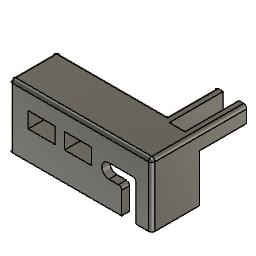
cordnew v7 (Autodesk Fusion 360 design; units mm, degrees)
Autodesk Fusion 360 part; units mm, degrees
sketch "Sketch1" plane through (0, 0, 0) normal (0, 1, 0) x (1, 0, 0)
  line L0 (0, 0) -> (90, 0)
  line L1 (90, 0) -> (90, -40)
  line L2 (90, -40) -> (0, -40)
  line L3 (0, -40) -> (0, 0)
  dimension "d1" = 90
  dimension "d2" = 40
  constraint horizontal L0
  constraint vertical L1
  constraint horizontal L2
  constraint vertical L3
  constraint coincident L0.start L3.end
  measures "d1" distance of L0.start L0.end
  measures "d2" distance of L0.end L1.end
extrude "Extrude1" add sketch "Sketch1" along normal blind 30
sketch "Sketch2" plane through (0, 30, 0) normal (0, 1, 0) x (-1, 0, 0)
  line L0 (0, 40) -> (-90, 40)
  line L1 (-90, 40) -> (-90, 0)
  line L2 (-90, 0) -> (0, 0)
  line L3 (0, 0) -> (0, 40)
  line L4 (-85, 0) -> (-5, 0)
  line L5 (-5, 0) -> (-5, 35)
  line L6 (-5, 35) -> (-85, 35)
  line L7 (-85, 35) -> (-85, 0)
  constraint horizontal L4
  constraint vertical L5
  constraint horizontal L6
  constraint vertical L7
  constraint coincident L2 L4.start
extrude "Extrude2" cut sketch "Sketch2" against normal blind 25 contours L2 L4 L5 L6 L7
sketch "Sketch3" plane through (0, 0, 0) normal (-1, 0, 0) x (0, -1, 0)
  line L0 (0, 0) -> (0, 40)
  line L1 (0, 40) -> (-30, 40)
  line L2 (-30, 40) -> (-30, 0)
  line L3 (-30, 0) -> (0, 0)
  line L4 (-25, 0) -> (-5, 0)
  line L5 (-5, 0) -> (-5, 10)
  line L6 (-5, 10) -> (-25, 10)
  line L7 (-25, 10) -> (-25, 0)
  constraint horizontal L4
  constraint vertical L5
  constraint horizontal L6
  constraint vertical L7
  constraint coincident L3 L4.start
extrude "Extrude3" cut sketch "Sketch3" against normal blind 5 contours L3 L4 L5 L6 L7
sketch "Sketch4" plane through (0, 30, 0) normal (0, 1, 0) x (-1, 0, 0)
  line L0 (-85, 0) -> (-85, 35)
  line L1 (-85, 35) -> (-5, 35)
  line L2 (-5, 35) -> (-5, 0)
  line L3 (-5, 0) -> (0, 0)
  line L4 (0, 0) -> (0, 40)
  line L5 (0, 40) -> (-90, 40)
  line L6 (-90, 40) -> (-90, 0)
  line L7 (-90, 0) -> (-85, 0)
  line L8 (-90, 40) -> (-70, 40)
  line L9 (-70, 40) -> (-70, 35)
  line L10 (-70, 35) -> (-90, 35)
  line L11 (-90, 35) -> (-90, 40)
  constraint horizontal L8
  constraint vertical L9
  constraint horizontal L10
  constraint vertical L11
  constraint coincident L5.end L6.start
extrude "Extrude4" add sketch "Sketch4" along normal blind 30 contours L1 L5 L6 L8 L9 L10 L11
sketch "Sketch5" plane through (0, 0, 40) normal (0, 0, 1) x (-1, 0, 0)
  line L0 (0, 0) -> (-90, 0)
  line L1 (-90, 0) -> (-90, -60)
  line L2 (-90, -60) -> (-70, -60)
  line L3 (-70, -60) -> (-70, -30)
  line L4 (-70, -30) -> (0, -30)
  line L5 (0, -30) -> (0, 0)
  line L6 (-75.0796, -60) -> (-85.0796, -60)
  line L7 (-85.0796, -60) -> (-85.0796, -26)
  line L8 (-85.0796, -26) -> (-75.0796, -26)
  line L9 (-75.0796, -26) -> (-75.0796, -60)
  dimension "d11" = 10
  dimension "d12" = 34
  constraint horizontal L6
  constraint vertical L7
  constraint horizontal L8
  constraint vertical L9
  constraint coincident L2 L6.start
  measures "d11" distance of L6.start L6.end
  measures "d12" distance of L6.end L7.end
extrude "Extrude5" cut sketch "Sketch5" against normal blind 5 contours L2 L6 L7 L8 L9
sketch "Sketch6" plane through (0, 5, 0) normal (0, 1, 0) x (-1, 0, 0)
  line L0 (-85, 35) -> (-85, 0)
  line L1 (-85, 0) -> (0, 0)
  line L2 (0, 0) -> (0, 10)
  line L3 (0, 10) -> (-5, 10)
  line L4 (-5, 10) -> (-5, 35)
  line L5 (-5, 35) -> (-85, 35)
  line L6 (-80, 25) -> (-71, 25)
  line L7 (-71, 16) -> (-71, 0)
  line L8 (-71, 0) -> (-80, 0)
  line L9 (-80, 0) -> (-80, 25)
  line L10 (-80, 25) -> (-63, 25)
  line L11 (-63, 16) -> (-71, 16)
  line L12 (-80, 16) -> (-80, 25)
  line L13 (-50, 28) -> (-33, 28)
  line L14 (-33, 28) -> (-33, 18)
  line L15 (-33, 18) -> (-50, 18)
  line L16 (-50, 18) -> (-50, 28)
  arc A0 (-63, 16) -> (-63, 25) centre (-63, 20.5) ccw
  dimension "d15" = 9
  dimension "d16" = 17
  constraint horizontal L6
  constraint vertical L7
  constraint horizontal L8
  constraint vertical L9
  constraint coincident L1 L7.end
  constraint horizontal L10
  constraint horizontal L11
  constraint vertical L12
  constraint horizontal L13
  constraint vertical L14
  constraint horizontal L15
  constraint vertical L16
  measures "d15" diameter of A0
  measures "d16" distance of L13.start L13.end
extrude "Extrude6" cut sketch "Sketch6" against normal blind 5 contours L1 L6 L7 L8 L9 L10 L11 L12 A0
sketch "Sketch7" plane through (0, 5, 0) normal (0, 1, 0) x (-1, 0, 0)
  line L0 (-80, 0) -> (-80, 25)
  line L1 (-80, 25) -> (-63, 25)
  arc A0 (-63, 16) -> (-63, 25) centre (-63, 20.5) ccw
  line L2 (-63, 16) -> (-71, 16)
  line L3 (-71, 16) -> (-71, 0)
  line L4 (-71, 0) -> (0, 0)
  line L5 (0, 0) -> (0, 10)
  line L6 (0, 10) -> (-5, 10)
  line L7 (-5, 10) -> (-5, 35)
  line L8 (-5, 35) -> (-85, 35)
  line L9 (-85, 35) -> (-85, 0)
  line L10 (-85, 0) -> (-80, 0)
  line L11 (-12, 28) -> (-29, 28)
  line L12 (-29, 28) -> (-29, 18)
  line L13 (-29, 18) -> (-12, 18)
  line L14 (-12, 18) -> (-12, 28)
  constraint horizontal L11
  constraint vertical L12
  constraint horizontal L13
  constraint vertical L14
extrude "Extrude7" cut sketch "Sketch7" against normal blind 8 contours L11 L12 L13 L14
sketch "Sketch8" plane through (0, 5, 0) normal (0, 1, 0) x (-1, 0, 0)
  line L0 (-29, 28) -> (-12, 28)
  line L1 (-12, 28) -> (-12, 18)
  line L2 (-12, 18) -> (-29, 18)
  line L3 (-29, 18) -> (-29, 28)
  line L4 (-80, 0) -> (-80, 25)
  line L5 (-80, 25) -> (-63, 25)
  arc A0 (-63, 16) -> (-63, 25) centre (-63, 20.5) ccw
  line L6 (-63, 16) -> (-71, 16)
  line L7 (-71, 16) -> (-71, 0)
  line L8 (-71, 0) -> (0, 0)
  line L9 (0, 0) -> (0, 10)
  line L10 (0, 10) -> (-5, 10)
  line L11 (-5, 10) -> (-5, 35)
  line L12 (-5, 35) -> (-85, 35)
  line L13 (-85, 35) -> (-85, 0)
  line L14 (-85, 0) -> (-80, 0)
  line L15 (-35, 28) -> (-52, 28)
  line L16 (-52, 28) -> (-52, 18)
  line L17 (-52, 18) -> (-35, 18)
  line L18 (-35, 18) -> (-35, 28)
  constraint horizontal L15
  constraint vertical L16
  constraint horizontal L17
  constraint vertical L18
extrude "Extrude8" cut sketch "Sketch8" against normal blind 6 contours L15 L16 L17 L18
sketch "Sketch9" plane through (0, 5, 0) normal (0, 1, 0) x (-1, 0, 0)
  line L0 (-52, 28) -> (-35, 28)
  line L1 (-35, 28) -> (-35, 18)
  line L2 (-35, 18) -> (-52, 18)
  line L3 (-52, 18) -> (-52, 28)
  line L4 (-29, 28) -> (-12, 28)
  line L5 (-12, 28) -> (-12, 18)
  line L6 (-12, 18) -> (-29, 18)
  line L7 (-29, 18) -> (-29, 28)
  line L8 (-80, 0) -> (-80, 25)
  line L9 (-80, 25) -> (-63, 25)
  arc A0 (-63, 16) -> (-63, 25) centre (-63, 20.5) ccw
  line L10 (-63, 16) -> (-71, 16)
  line L11 (-71, 16) -> (-71, 0)
  line L12 (-71, 0) -> (0, 0)
  line L13 (0, 0) -> (0, 10)
  line L14 (0, 10) -> (-5, 10)
  line L15 (-5, 10) -> (-5, 35)
  line L16 (-5, 35) -> (-85, 35)
  line L17 (-85, 35) -> (-85, 0)
  line L18 (-85, 0) -> (-80, 0)
  line L19 (-54, 30) -> (-33, 30)
  line L20 (-33, 30) -> (-33, 15)
  line L21 (-33, 15) -> (-54, 15)
  line L22 (-54, 15) -> (-54, 30)
  constraint horizontal L19
  constraint vertical L20
  constraint horizontal L21
  constraint vertical L22
extrude "Extrude9" add sketch "Sketch9" along normal blind 20 contours L19 L20 L21 L22
sketch "Sketch10" plane through (0, 5, 0) normal (0, 1, 0) x (-1, 0, 0)
  line L0 (-54, 15) -> (-54, 30)
  line L1 (-54, 30) -> (-33, 30)
  line L2 (-33, 30) -> (-33, 15)
  line L3 (-33, 15) -> (-54, 15)
  line L4 (-29, 28) -> (-12, 28)
  line L5 (-12, 28) -> (-12, 18)
  line L6 (-12, 18) -> (-29, 18)
  line L7 (-29, 18) -> (-29, 28)
  line L8 (-80, 0) -> (-80, 25)
  line L9 (-80, 25) -> (-63, 25)
  arc A0 (-63, 16) -> (-63, 25) centre (-63, 20.5) ccw
  line L10 (-63, 16) -> (-71, 16)
  line L11 (-71, 16) -> (-71, 0)
  line L12 (-71, 0) -> (0, 0)
  line L13 (0, 0) -> (0, 10)
  line L14 (0, 10) -> (-5, 10)
  line L15 (-5, 10) -> (-5, 35)
  line L16 (-5, 35) -> (-85, 35)
  line L17 (-85, 35) -> (-85, 0)
  line L18 (-85, 0) -> (-80, 0)
  line L19 (-31, 30) -> (-10, 30)
  line L20 (-10, 30) -> (-10, 15)
  line L21 (-10, 15) -> (-31, 15)
  line L22 (-31, 15) -> (-31, 30)
  constraint horizontal L19
  constraint vertical L20
  constraint horizontal L21
  constraint vertical L22
extrude "Extrude10" add sketch "Sketch10" along normal blind 20 contours L19 L20 L21 L22
sketch "Sketch11" plane through (0, 0, 0) normal (-1, 0, 0) x (0, -1, 0)
  line L0 (-25, 0) -> (-25, 10)
  line L1 (-25, 10) -> (-5, 10)
  line L2 (-5, 10) -> (-5, 0)
  line L3 (-5, 0) -> (0, 0)
  line L4 (0, 0) -> (0, 40)
  line L5 (0, 40) -> (-30, 40)
  line L6 (-30, 40) -> (-30, 0)
  line L7 (-30, 0) -> (-25, 0)
  line L8 (-25, 0) -> (-30, 0)
  line L9 (-30, 0) -> (-30, 18)
  line L10 (-30, 18) -> (-25, 18)
  line L11 (-25, 18) -> (-25, 0)
  dimension "d27" = 18
  constraint horizontal L8
  constraint vertical L9
  constraint horizontal L10
  constraint vertical L11
  constraint coincident L6 L9.end
  constraint coincident L0.start L7.end
  measures "d27" distance of L6.end L9.end
extrude "Extrude11" add sketch "Sketch11" against normal blind 54 contours L0 L6 L7 L8 L9 L10 L11
sketch "Sketch12" plane through (0, 0, 15) normal (0, 0, -1) x (1, 0, 0)
  line L0 (54, -5) -> (33, -5)
  line L1 (33, -5) -> (33, -25)
  line L2 (33, -25) -> (54, -25)
  line L3 (54, -25) -> (54, -5)
  circle A0 centre (43.5, -17.5) radius 1.5
  circle A1 centre (20, -17.5) radius 1.5
  line L4 (54, -25) -> (0, -25)
  dimension "d30" = 7.5
  dimension "d31" = 3
  dimension "d32" = 7.5
  dimension "d33" = 3
  measures "d30" distance of L2 A0.centre
  measures "d31" diameter of A0
  measures "d32" distance of A1.centre L4
  measures "d33" diameter of A1
extrude "Extrude12" cut sketch "Sketch12" against normal blind 4 contours A0
sketch "Sketch13" plane through (0, 0, 15) normal (0, 0, -1) x (1, 0, 0)
  line L0 (31, -5) -> (10, -5)
  line L1 (10, -5) -> (10, -25)
  line L2 (10, -25) -> (31, -25)
  line L3 (31, -25) -> (31, -5)
  circle A0 centre (20, -17.5) radius 1.5
  dimension "d36" = 7.5
  dimension "d37" = 3
  dimension "d38" = 11
  measures "d36" distance of L2 A0.centre
  measures "d37" diameter of A0
  measures "d38" distance of L3 A0.centre
extrude "Extrude13" cut sketch "Sketch13" against normal blind 4 contours A0
sketch "Sketch14" plane through (0, 30, 0) normal (0, 1, 0) x (-1, 0, 0)
  line L0 (0, 0) -> (0, 40)
  line L1 (0, 40) -> (-70, 40)
  line L2 (-70, 40) -> (-70, 35)
  line L3 (-70, 35) -> (-5, 35)
  line L4 (-5, 35) -> (-5, 18)
  line L5 (-5, 18) -> (-54, 18)
  line L6 (-54, 18) -> (-54, 0)
  line L7 (-54, 0) -> (0, 0)
  line L8 (-54, 10) -> (-31, 10)
  line L9 (-31, 10) -> (-31, 0)
  line L10 (-31, 0) -> (-54, 0)
  line L11 (-54, 0) -> (-54, 10)
  dimension "d41" = 10
  constraint horizontal L8
  constraint vertical L9
  constraint horizontal L10
  constraint vertical L11
  constraint coincident L7 L9.end
  constraint coincident L6 L8.start
  measures "d41" distance of L8.start L6.end
extrude "Extrude14" cut sketch "Sketch14" against normal blind 5 contours L6 L7 L8 L9 L10 L11
sketch "Sketch15" plane through (0, 0, 35) normal (0, 0, -1) x (1, 0, 0)
  line L0 (75.0796, -26) -> (85, -26)
  line L1 (85, -26) -> (85, -5)
  line L2 (85, -5) -> (5, -5)
  line L3 (5, -5) -> (5, -30)
  line L4 (5, -30) -> (70, -30)
  line L5 (70, -30) -> (70, -60)
  line L6 (70, -60) -> (75.0796, -60)
  line L7 (75.0796, -60) -> (75.0796, -26)
  line L8 (75.0796, -26) -> (70, -26)
  line L9 (70, -26) -> (70, -60)
  line L10 (70, -60) -> (75.0796, -60)
  line L11 (75.0796, -60) -> (75.0796, -26)
  constraint horizontal L8
  constraint vertical L9
  constraint horizontal L10
  constraint vertical L11
  constraint coincident L5.end L6.start
  constraint coincident L0.start L7.end
extrude "Extrude15" add sketch "Sketch15" along normal blind 5 contours L5 L6 L7 L8 L9 L10 L11
extrude "Extrude16" add 1 faces at (88.3599, 50, 35) along direction (0, 0, -1) blind 5
sketch "Sketch16" plane through (0, 60, 0) normal (0, 1, 0) x (-1, 0, 0)
  line L0 (-85.0796, 30) -> (-85.0796, 40)
  line L1 (-85.0796, 40) -> (-90, 40)
  line L2 (-90, 40) -> (-90, 30)
  line L3 (-90, 30) -> (-85.0796, 30)
sketch "Sketch17" plane through (0, 0, 30) normal (0, 0, -1) x (1, 0, 0)
  line L0 (75.0796, -60) -> (75.0796, -26)
  line L1 (75.0796, -26) -> (70, -26)
  line L2 (70, -26) -> (70, -60)
  line L3 (70, -60) -> (75.0796, -60)
  line L4 (75.0796, -26) -> (70, -26)
  line L5 (70, -26) -> (70, -21)
  line L6 (70, -21) -> (75.0796, -21)
  line L7 (75.0796, -21) -> (75.0796, -26)
  constraint horizontal L4
  constraint vertical L5
  constraint horizontal L6
  constraint vertical L7
  constraint coincident L0.end L1.start
extrude "Extrude17" add sketch "Sketch17" against normal blind 5 contours L1 L4 L5 L6 L7
fillet "Fillet1" radius 2 1 edges at (90, 0, 20)
fillet "Fillet2" radius 2 3 edges at (90, 31, 40) (89.4142, 0.5858, 40) (44, 0, 40)
fillet "Fillet3" radius 2 3 edges at (0, 16, 40) (0, 0.5858, 39.4142) (0, 0, 19)
fillet "Fillet4" radius 2 3 edges at (0, 30, 19) (0.5858, 30, 39.4142) (36, 30, 40)
fillet "Fillet5" radius 2 1 edges at (70, 44, 40)
fillet "Fillet6" radius 2 1 edges at (80, 2.5, 25)
fillet "Fillet7" radius 2 1 edges at (71, 2.5, 16)
